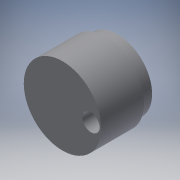
# Autodesk Inventor part: RotationDisk
Saved by Autodesk Inventor 2016 (Build 200138000, 138)
## iProperties
Created: 2017-02-18
Part Number: RotationDisk
Material: Generic
Document SubType Name: Modeling
Designer: Owner
Density: 1 g/cm^3
Appearance: Default
Author: Owner
Autodesk Inventor part; units mm, degrees
ref_plane "YZ Plane" through (0, 0, 0) normal (1, 0, 0) x (0, 1, 0)
ref_plane "XZ Plane" through (0, 0, 0) normal (0, 1, 0) x (-1, 0, 0)
ref_plane "XY Plane" through (0, 0, 0) normal (0, 0, 1) x (1, 0, 0)
sketch "Sketch1" plane through (0, 0, 0) normal (0, 0, 1) x (1, 0, 0)
  circle A0 centre (0, 0) radius 9.5
  arc A1 (-3.096, -4.5458) -> (5.2116, 1.7576) centre (0, 0) ccw projected
  point P0 (0, 0)
  dimension "d0" = 19
  constraints: 1 centre point
  measures "d0" diameter of A0
extrude "Extrusion1" add sketch "Sketch1" along normal blind 10.5
sketch "Sketch2" plane through (0, 0, 10.5) normal (0, 0, 1) x (1, 0, 0)
  circle A0 centre (0, 0) radius 9.5 projected
  line L0 (9.5, 0) -> (7, 0)
  circle A1 centre (7, 0) radius 2.125
  point P0 (0, 0)
  dimension "d3" = 2.5
  dimension "d4" = 4.25
  constraints: 2 end point, 1 centre point, 1 coincident, 1 horizontal, 1 horizontal alignment, 1 other
  measures "d3" distance of L0.start L0.end
  measures "d4" diameter of A1
extrude "Extrusion2" cut sketch "Sketch2" against normal blind 5 contours A1
sketch "Sketch3" plane through (0, 0, 0) normal (0, 0, -1) x (-1, 0, 0)
  circle A0 centre (0, 0) radius 5 projected
  circle A1 centre (0, 0) radius 9.5 projected
  circle A2 centre (0, 0) radius 8.5
  point P0 (0, 0)
  dimension "d7" = 17
  constraints: 1 centre point, 1 coincident
  measures "d7" diameter of A2
extrude "Extrusion3" add sketch "Sketch3" along normal blind 3 contours A0 | A2
body "Solid1"
